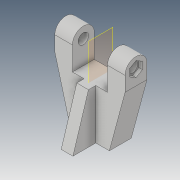
# Autodesk Inventor part: Camera Holder
Saved by Autodesk Inventor 2018 (Build 220112000, 112)
## iProperties
Created: 2018-10-15
Part Number: Camera Holder
Material: Generic
Document SubType Name: Modeling
Designer: Micah
Density: 1 g/cm^3
Appearance: Default
Author: Micah
Autodesk Inventor part; units mm, degrees
ref_plane "YZ Plane" through (0, 0, 0) normal (1, 0, 0) x (0, 1, 0)
ref_plane "XZ Plane" through (0, 0, 0) normal (0, 1, 0) x (-1, 0, 0)
ref_plane "XY Plane" through (0, 0, 0) normal (0, 0, 1) x (1, 0, 0)
sketch "Sketch1" plane through (0, 0, 0) normal (1, 0, 0) x (0, 1, 0)
  circle A0 centre (0, 0) radius 2.25
  circle A1 centre (0, 0) radius 4.75
  line L0 (0, 4.75) -> (-10.16, 4.75)
  line L1 (0, -4.75) -> (-10.16, -4.75)
  line L2 (-10.16, 4.75) -> (-10.16, -4.75)
  dimension "d0" = 4.5
  dimension "d1" = 9.5
  dimension "d2" = 10.16
  dimension "d3" = 10.16
  constraints: 6 end point, 2 centre point, 2 coincident, 2 horizontal, 2 point on circle, 2 tangent
  measures "d0" diameter of A0
  measures "d1" diameter of A1
  measures "d2" horizontal distance of point (0, 0) L0.end
  measures "d3" distance of L1.start L1.end
extrude "Extrusion1" add sketch "Sketch1" along normal blind 7.62
ref_plane "Work Plane1" through (15.24, 0, 0) normal (1, 0, 0) x (0, 0, -1)
mirror "Mirror1" about plane through (15.24, 0, 0) normal (1, 0, 0) of "Extrusion1"
sketch "Sketch2" plane through (30.48, -10.16, 4.75) normal (1, 0, 0) x (0, 0, -1)
  circle A0 centre (4.75, 10.16) radius 2.25 projected
  line L0 (7.5, 8.5723) -> (4.75, 6.9846)
  line L1 (4.75, 6.9846) -> (2, 8.5723)
  line L2 (2, 8.5723) -> (2, 11.7477)
  line L3 (2, 11.7477) -> (4.75, 13.3354)
  line L4 (4.75, 13.3354) -> (7.5, 11.7477)
  line L5 (7.5, 11.7477) -> (7.5, 8.5723)
  dimension "d7" = 5.5
  constraints: 12 end point, 1 coincident, 13 other
  measures "d7" distance between parallel lines of L5 L2
extrude "Extrusion2" cut sketch "Sketch2" against normal blind 1.5
sketch "Sketch3" plane through (0, 0, 0) normal (-1, 0, 0) x (0, 0, 1)
  circle A0 centre (0, 0) radius 2.75
  dimension "d10" = 5.5
  constraints: 1 centre point, 1 coincident
  measures "d10" diameter of A0
extrude "Extrusion3" cut sketch "Sketch3" against normal blind 1.5
sketch "Sketch4" plane through (0, 0, 0) normal (-1, 0, 0) x (0, 0, 1)
  line L0 (4.75, 0) -> (7.925, -10.16)
  line L1 (4.75, -10.16) -> (-4.75, -10.16) projected
  line L2 (7.925, -10.16) -> (4.75, -10.16)
  line L3 (4.75, 0) -> (4.75, -10.16)
  point P0 (0, 0)
  dimension "d13" = 3.175
  constraints: 6 end point, 1 collinear, 1 vertical
  measures "d13" distance of L0.end L1.start
extrude "Extrusion4" add sketch "Sketch4" against normal up to surface (30.48 mm away)
sketch "Sketch5" plane through (0, 0, 0) normal (-1, 0, 0) x (0, 0, 1)
  line L0 (-4.75, -10.16) -> (-4.75, 0) projected
  line L1 (-4.75, -10.16) -> (-4.75, -31.75)
  line L2 (4.75, 0) -> (4.75, -10.16) projected
  line L3 (7.925, -10.16) -> (14.6719, -31.75)
  line L4 (4.75, 0) -> (7.925, -10.16) projected
  line L5 (-4.75, -31.75) -> (14.6719, -31.75)
  line L6 (7.925, -10.16) -> (-4.75, -10.16) projected
  line L7 (-4.75, -10.16) -> (7.925, -10.16)
  point P0 (0, 0)
  dimension "d16" = 31.75
  constraints: 8 end point, 2 collinear, 1 horizontal, 1 point on line, 1 vertical
  measures "d16" vertical distance of L1.end point (0, 0)
extrude "Extrusion5" add sketch "Sketch5" against normal up to surface (30.48 mm away) contours L6 L3 L5 L1
sketch "Sketch6" plane through (7.62, 0, -4.75) normal (0, 0, -1) x (-1, 0, 0)
  line L0 (-22.86, -31.75) -> (-22.86, 0) projected
  line L1 (-22.86, -6.35) -> (-16.0541, -31.75)
  line L2 (7.62, -31.75) -> (-22.86, -31.75) projected
  line L3 (7.62, -6.35) -> (0.8141, -31.75)
  line L4 (7.62, 0) -> (7.62, -31.75) projected
  line L5 (-22.86, -6.35) -> (-22.86, -31.75)
  line L6 (-22.86, -31.75) -> (-16.0541, -31.75)
  line L7 (0.8141, -31.75) -> (7.62, -31.75)
  line L8 (7.62, -6.35) -> (7.62, -31.75)
  dimension "d20" = 15
  dimension "d21" = 6.35
  dimension "d22" = 15
  dimension "d23" = 6.35
  constraints: 12 end point, 4 point on line, 3 collinear, 1 horizontal
  measures "d20" angle of L0 L1
  measures "d21" distance of L0.end L1.start
  measures "d22" angle of L4 L3
  measures "d23" distance of L4.start L3.start
extrude "Extrusion6" cut sketch "Sketch6" against normal through all
sketch "Sketch7" plane through (6.8059, -31.75, 14.6719) normal (0, -1, 0) x (1, 0, 0)
  line L0 (16.0541, -12.4219) -> (16.0541, -16.9219) projected
  line L1 (16.0541, -19.4219) -> (16.0541, -9.9219) projected
  line L2 (16.0541, -9.9219) -> (16.0541, -19.4219) projected
  line L3 (0.8141, -12.4219) -> (0.8141, -16.9219) projected
  line L4 (0.8141, -9.9219) -> (0.8141, -19.4219) projected
  line L5 (0.8141, -19.4219) -> (0.8141, -9.9219) projected
  line L6 (0.8141, -19.4219) -> (0.8141, -9.9219) projected
  line L7 (0, 0) -> (16.8682, 0) projected
  line L8 (5.8941, 0) -> (10.9741, 0)
  line L9 (10.9741, 0) -> (10.9741, -9.9219)
  line L10 (10.9741, -9.9219) -> (5.8941, -9.9219)
  line L11 (5.8941, -9.9219) -> (5.8941, 0)
  line L12 (5.8941, -9.9219) -> (-12.9487, -9.9219)
  line L13 (-12.9487, -9.9219) -> (-12.9487, 3.2333)
  line L14 (-12.9487, 3.2333) -> (5.8941, 3.2333)
  line L15 (5.8941, 3.2333) -> (5.8941, -9.9219)
  line L16 (10.9741, -9.9219) -> (26.322, -9.9219)
  line L17 (26.322, -9.9219) -> (26.322, 1.6077)
  line L18 (26.322, 1.6077) -> (10.9741, 1.6077)
  line L19 (10.9741, 1.6077) -> (10.9741, -9.9219)
  point P0 (-6.8059, -14.6719)
  dimension "d28" = 5.08
  dimension "d29" = 0
  dimension "d30" = 5.8941
  dimension "d31" = 5.8941
  constraints: 24 end point, 6 parallel, 3 horizontal, 3 perpendicular, 1 point on line
  measures "d28" distance between parallel lines of L11 L9
  measures "d29" distance from line of L2.start L10
  measures "d30" distance from line of L7.end L9
  measures "d31" distance of L7.start L8.start
extrude "Extrusion7" cut sketch "Sketch7" against normal through all contours L11 L12 L13 L14 L15 | L19 L18 L17 L16 L9
sketch "Sketch8" plane through (17.78, -31.75, 14.6719) normal (1, 0, 0) x (0, 0, -1)
  line L0 (9.9219, 21.59) -> (19.4219, 21.59) projected
  line L1 (9.9219, 21.59) -> (19.4219, 21.59) projected
  line L2 (9.9219, 21.59) -> (5.1304, 21.59)
  line L3 (5.1304, 21.59) -> (9.9219, 31.75)
  line L4 (9.9219, 31.75) -> (9.9219, 21.59)
  line L5 (9.9219, 0) -> (9.9219, 25.4) projected
  point P0 (14.6719, 31.75)
  constraints: 6 end point, 1 collinear, 1 horizontal
extrude "Extrusion8" cut sketch "Sketch8" against normal up to surface (5.08 mm away)
equation "\"d30\" = d31"
body "Solid1"
